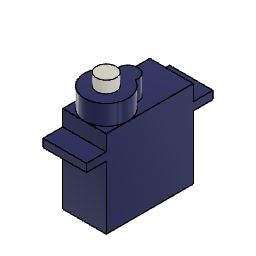
Savöx_SH_0255 MG_micro_servo (Autodesk Fusion 360 design; units mm, degrees)
Autodesk Fusion 360 part; units mm, degrees
sketch "Servo Side Profile" plane through (0, 0, 0) normal (1, 0, 0) x (0, 1, 0)
  line L0 (0, 0) -> (22, 0)
  line L1 (22, 0) -> (22, 16)
  line L2 (22, 16) -> (27, 16)
  line L3 (27, 16) -> (27, 18)
  line L4 (27, 18) -> (22, 18)
  line L5 (22, 18) -> (22, 22)
  line L6 (22, 22) -> (0, 22)
  line L7 (0, 22) -> (0, 18)
  line L8 (0, 18) -> (-5, 18)
  line L9 (-5, 18) -> (-5, 16)
  line L10 (-5, 16) -> (0, 16)
  line L11 (0, 16) -> (0, 0)
  dimension "d1" = 22
  dimension "d2" = 22
  dimension "d3" = 16
  dimension "d4" = 16
  dimension "d5" = 2
  dimension "d6" = 2
  dimension "d7" = 4
  dimension "d9" = 5
  dimension "d10" = 5
  constraint coincident L0.start L11.end
  constraint horizontal L0
  constraint perpendicular L0 L1
  constraint perpendicular L1 L2
  constraint perpendicular L2 L3
  constraint perpendicular L3 L4
  constraint perpendicular L4 L5
  constraint perpendicular L3 L6
  constraint perpendicular L6 L7
  constraint perpendicular L3 L8
  constraint perpendicular L8 L9
  constraint perpendicular L9 L10
  constraint perpendicular L0 L11
  constraint collinear L7 L11
  measures "d1" distance of L0.start L0.end
  measures "d2" distance of L5.end L6.end
  measures "d3" distance of L0.end L1.end
  measures "d4" distance of L10.end L0.start
  measures "d5" distance of L2.end L3.end
  measures "d6" distance of L8.end L9.end
  measures "d7" distance of L6.end L7.end
  measures "d9" distance of L3.end L4.end
  measures "d10" distance of L7.end L8.end
extrude "Extrude1" add sketch "Servo Side Profile" along normal blind 11 makes body 1
sketch "Top Cylinders" plane through (0, 0, 22) normal (0, 0, 1) x (-1, 0, 0)
  line L0 (0, -22) -> (0, 0)
  line L1 (0, 0) -> (-11, 0)
  line L2 (-11, 0) -> (-11, -22)
  line L3 (-11, -22) -> (0, -22)
  circle A0 centre (-5.5, -5.5) radius 5.5
  circle A1 centre (-5.5, -11) radius 2.5
  dimension "d13" = 5.5
  dimension "d14" = 5.5
  dimension "d15" = 11
  dimension "d16" = 5.5
  dimension "d17" = 11
  dimension "d18" = 5
  measures "d13" distance of L2 A0.centre
  measures "d14" distance of L1 A0.centre
  measures "d15" diameter of A0
  measures "d16" distance of L2 A1.centre
  measures "d17" distance of L1 A1.centre
  measures "d18" diameter of A1
extrude "Extrude2" add sketch "Top Cylinders" along normal blind 5 contours A0 A1 | A0 A1 | A0 A1 bodies 1
sketch "Turning Gear" plane through (0, 0, 27) normal (0, 0, 1) x (-1, 0, 0)
  arc A0 (-7.9346, -10.4318) -> (-3.0654, -10.4318) centre (-5.5, -11) ccw
  arc A1 (-3.0654, -10.4318) -> (-7.9346, -10.4318) centre (-5.5, -5.5) ccw
  circle A2 centre (-5.5, -5.5) radius 2.5
  dimension "d21" = 5
  constraint concentric A1 A2
  measures "d21" diameter of A2
extrude "Extrude3" add sketch "Turning Gear" along normal blind 3 separate body contours A2 makes body 2
equation "d13 = ( 11 / 2 ) * 1 mm"
equation "d14 = ( 11 / 2 ) * 1 mm"
equation "d16 = ( 11 / 2 ) * 1 mm"
equation "d17 = ( 22 / 2 ) * 1 mm"
named bodies: "Servo Motor Body", "Turning Gear"
